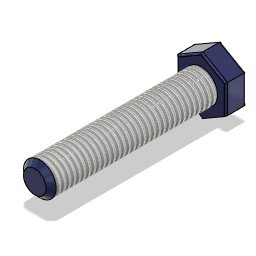
0.163.0902 - Vis H - M12-50_30 (Autodesk Fusion 360 design; units mm, degrees)
Autodesk Fusion 360 part; units mm, degrees
sketch "Sketch1" plane through (0, 0, 0) normal (0, 0, 1) x (1, 0, 0)
  circle A0 centre (0, 0) radius 6
  dimension "d1" = 12
  constraint coincident A0.centre origin
  measures "d1" diameter of A0
extrude "Extrude1" add sketch "Sketch1" along normal blind 50
thread "Thread1" "ISO Metric profile 10.0 M10x1.5 6g" major diameter 9.85 minor diameter 8.141 pitch 1.5 angle 60 resizes the face on face at (5.9702, -0.5974, 16.6667)
sketch "Sketch2" plane through (0, 0, 0) normal (0, 0, -1) x (-1, 0, 0)
  circle A0 centre (0, 0) radius 4.925
  line L0 (4.925, 2.8435) -> (0, 5.6869) construction
  line L1 (0, 5.6869) -> (-4.925, 2.8435) construction
  line L2 (-4.925, 2.8435) -> (-4.925, -2.8435) construction
  line L3 (-4.925, -2.8435) -> (0, -5.6869) construction
  line L4 (0, -5.6869) -> (4.925, -2.8435) construction
  line L5 (4.925, -2.8435) -> (4.925, 2.8435) construction
  line L6 (0, 8.5737) -> (-7.425, 4.2868)
  line L7 (-7.425, 4.2868) -> (-7.425, -4.2868)
  line L8 (-7.425, -4.2868) -> (0, -8.5737)
  line L9 (0, -8.5737) -> (7.425, -4.2868)
  line L10 (7.425, -4.2868) -> (7.425, 4.2868)
  line L11 (7.425, 4.2868) -> (0, 8.5737)
  dimension "d4" = 2.5
  constraint coincident A0.centre origin
extrude "Extrude2" add sketch "Sketch2" along normal blind 6 contours A0 | L6 L7 L8 L9 L10 L11
fillet "Fillet1" radius 0.5 11 edges at (3.7125, -6.4302, -6) (-3.7125, -6.4302, -6) (-7.425, 0, -6) (-3.7125, 6.4302, -6) (3.7125, 6.4302, -6) (7.425, 0, -6) (-3.7125, -6.4302, 0) (-7.425, 0, 0) (-3.7125, 6.4302, 0) (3.7125, 6.4302, 0) (7.425, 0, 0)
chamfer "Chamfer1" distance 1.5 angle 45 1 edges at (-4.5917, -1.781, 50)
